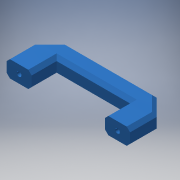
# Autodesk Inventor part: FrameHandle
Saved by Autodesk Inventor 2016 (Build 200138000, 138)
## iProperties
Category: Print
Created: 2015-04-26
Part Number: FrameHandle
Material: ABS Plastic
Document SubType Name: Modeling
Designer: Jack
Density: 1.06 g/cm^3
Appearance: Cyan
Author: Jack
Title: Frame Handle
Autodesk Inventor part; units mm, degrees
ref_plane "YZ Plane" through (0, 0, 0) normal (1, 0, 0) x (0, 1, 0)
ref_plane "XZ Plane" through (0, 0, 0) normal (0, 1, 0) x (-1, 0, 0)
ref_plane "XY Plane" through (0, 0, 0) normal (0, 0, 1) x (1, 0, 0)
sketch "Sketch1" plane through (0, 0, 0) normal (0, 0, 1) x (1, 0, 0)
  line L0 (0, 0) -> (0, 52)
  line L1 (0, 52) -> (148, 52)
  line L2 (148, 52) -> (148, 0)
  line L3 (148, 0) -> (118, 0)
  line L4 (118, 0) -> (118, 30)
  line L5 (118, 30) -> (30, 30)
  line L6 (30, 30) -> (30, 0)
  line L7 (30, 0) -> (0, 0)
  dimension "d0" = 52
  dimension "d1" = 88
  dimension "d2" = 30
  dimension "d3" = 30
  constraints: 16 end point, 7 perpendicular, 1 collinear, 1 point on line, 1 vertical
  measures "d0" distance of L0.start L0.end
  measures "d1" distance between parallel lines of L4 L6
  measures "d2" distance of L2.end L3.end
  measures "d3" distance of L5.end L6.end
extrude "Extrusion1" add sketch "Sketch1" along normal blind 20
chamfer "Chamfer1" distance 20 angle 45 2 edges at (0, 52, 10) (148, 52, 10)
sketch "Sketch3" plane through (20, 52, 0) normal (0, 1, 0) x (1, 0, 0)
  line L0 (-20, -20) -> (0, -20) projected
  line L1 (0, -20) -> (0, 0) projected
  line L2 (0, 0) -> (-20, 0) projected
  line L3 (-20, 0) -> (-20, -20) projected
  line L4 (108, -20) -> (128, -20) projected
  line L5 (128, -20) -> (128, 0) projected
  line L6 (128, 0) -> (108, 0) projected
  line L7 (108, 0) -> (108, -20) projected
  line L8 (10, 0) -> (-20, 0) projected
  line L9 (10, 0) -> (10, -20) projected
  line L10 (-20, -20) -> (10, -20) projected
  line L11 (-20, 0) -> (-20, -20) projected
  line L12 (128, 0) -> (98, 0) projected
  line L13 (128, 0) -> (128, -20) projected
  line L14 (98, -20) -> (128, -20) projected
  line L15 (98, 0) -> (98, -20) projected
  point P0 (-5, -10)
  point P1 (113, -10)
  dimension "d25" = 15
  dimension "d26" = 10
  dimension "d27" = 15
  constraints: 1 horizontal alignment
  measures "d25" distance from line of L5 point (113, -10)
  measures "d26" distance from line of L4 point (113, -10)
  measures "d27" distance from line of L3 point (-5, -10)
hole "Hole2" at (15, 52, 10) at (133, 52, 10) direction (0, -1, 0) diameter 5.5 end through all counterbore diameter 9 counterbore depth 40
chamfer "Chamfer3" distance 4 angle 45 16 edges at (74, 52, 20) (10, 42, 20) (0, 16, 20) (138, 42, 20) (148, 16, 20) (138, 42, 0) (148, 16, 0) (74, 52, 0) (10, 42, 0) (0, 16, 0) (30, 15, 0) (74, 30, 0) (118, 15, 0) (74, 30, 20) (30, 15, 20) (118, 15, 20)
body "Solid1"
